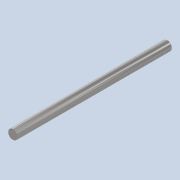
# Autodesk Inventor part: 0005-10-1006 Bara rectificata
Saved by Autodesk Inventor 2020 (Build 240168000, 168)
## iProperties
Created: 2020-12-18
Part Number: 0005-10-1006 Bara rectificata
Material: Stainless Steel
Document SubType Name: Modeling
Designer: Iulian Bors
Density: 8 g/cm^3
Appearance: Semi-Polished
Mass: 104.24 g
Surface Area: 53.5307 cm^2
Volume: 13.03 cm^3
Author: Iulian Bors
Subject: 10-1006
Autodesk Inventor part; units mm, degrees
ref_plane "YZ Plane" through (0, 0, 0) normal (1, 0, 0) x (0, 1, 0)
ref_plane "XZ Plane" through (0, 0, 0) normal (0, 1, 0) x (-1, 0, 0)
ref_plane "XY Plane" through (0, 0, 0) normal (0, 0, 1) x (1, 0, 0)
sketch "Sketch1" plane through (0, 0, 0) normal (0, 0, 1) x (1, 0, 0)
  circle A0 centre (0, 0) radius 5
  dimension "d0" = 10
  constraints: 1 centre point, 1 coincident
  measures "d0" diameter of A0
extrude "Extrusion1" add sketch "Sketch1" along normal blind 166
chamfer "Chamfer1" distance 0.5 angle 45 2 edges at (-5, 0, 166) (-5, 0, 0)
body "Solid1"
